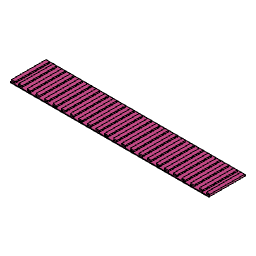
0_15m_Joch_Gerade_Schablone (Autodesk Fusion 360 design; units mm, degrees)
Autodesk Fusion 360 part; units mm, degrees
sketch "Skizze1" plane through (0, 0, 0) normal (0, 0, 1) x (1, 0, 0)
  line L0 (-3, 29.1) -> (3, 29.1)
  line L1 (3, 29.1) -> (3, 0)
  line L2 (3, 0) -> (-3, 0)
  line L3 (-3, 0) -> (-3, 29.1)
  line L4 (0, 29.1) -> (0, 0) construction
  line L5 (0, 0) -> (500, 0) construction
  line L6 (9.1, 29.1) -> (15.1, 29.1)
  line L7 (15.1, 29.1) -> (15.1, 0)
  line L8 (15.1, 0) -> (9.1, 0)
  line L9 (9.1, 0) -> (9.1, 29.1)
  line L10 (12.1, 29.1) -> (12.1, 0) construction
  line L11 (26.5, 29.1) -> (26.5, 0) construction
  line L12 (23.5, 29.1) -> (29.5, 29.1)
  line L13 (29.5, 0) -> (23.5, 0)
  line L14 (23.5, 0) -> (23.5, 29.1)
  line L15 (29.5, 29.1) -> (29.5, 0)
  line L16 (58.3, 0) -> (52.3, 0)
  line L17 (55.3, 29.1) -> (55.3, 0) construction
  line L18 (43.9, 29.1) -> (43.9, 0)
  line L19 (37.9, 29.1) -> (43.9, 29.1)
  line L20 (52.3, 29.1) -> (58.3, 29.1)
  line L21 (58.3, 29.1) -> (58.3, 0)
  line L22 (40.9, 29.1) -> (40.9, 0) construction
  line L23 (43.9, 0) -> (37.9, 0)
  line L24 (52.3, 0) -> (52.3, 29.1)
  line L25 (37.9, 0) -> (37.9, 29.1)
  line L26 (84.1, 29.1) -> (84.1, 0) construction
  line L27 (66.7, 0) -> (66.7, 29.1)
  line L28 (69.7, 29.1) -> (69.7, 0) construction
  line L29 (95.5, 0) -> (95.5, 29.1)
  line L30 (98.5, 29.1) -> (98.5, 0) construction
  line L31 (66.7, 29.1) -> (72.7, 29.1)
  line L32 (81.1, 0) -> (81.1, 29.1)
  line L33 (72.7, 29.1) -> (72.7, 0)
  line L34 (101.5, 29.1) -> (101.5, 0)
  line L35 (95.5, 29.1) -> (101.5, 29.1)
  line L36 (109.9, 29.1) -> (115.9, 29.1)
  line L37 (72.7, 0) -> (66.7, 0)
  line L38 (87.1, 0) -> (81.1, 0)
  line L39 (109.9, 0) -> (109.9, 29.1)
  line L40 (115.9, 0) -> (109.9, 0)
  line L41 (115.9, 29.1) -> (115.9, 0)
  line L42 (112.9, 29.1) -> (112.9, 0) construction
  line L43 (81.1, 29.1) -> (87.1, 29.1)
  line L44 (87.1, 29.1) -> (87.1, 0)
  line L45 (101.5, 0) -> (95.5, 0)
  line L46 (156.1, 29.1) -> (156.1, 0) construction
  line L47 (144.7, 29.1) -> (144.7, 0)
  line L48 (153.1, 29.1) -> (159.1, 29.1)
  line L49 (138.7, 29.1) -> (144.7, 29.1)
  line L50 (153.1, 0) -> (153.1, 29.1)
  line L51 (167.5, 29.1) -> (173.5, 29.1)
  line L52 (196.3, 0) -> (196.3, 29.1)
  line L53 (202.3, 0) -> (196.3, 0)
  line L54 (216.7, 0) -> (210.7, 0)
  line L55 (130.3, 29.1) -> (130.3, 0)
  line L56 (130.3, 0) -> (124.3, 0)
  line L57 (181.9, 29.1) -> (187.9, 29.1)
  line L58 (173.5, 29.1) -> (173.5, 0)
  line L59 (124.3, 0) -> (124.3, 29.1)
  line L60 (144.7, 0) -> (138.7, 0)
  line L61 (210.7, 0) -> (210.7, 29.1)
  line L62 (225.1, 29.1) -> (231.1, 29.1)
  line L63 (127.3, 29.1) -> (127.3, 0) construction
  line L64 (159.1, 29.1) -> (159.1, 0)
  line L65 (210.7, 29.1) -> (216.7, 29.1)
  line L66 (187.9, 0) -> (181.9, 0)
  line L67 (216.7, 29.1) -> (216.7, 0)
  line L68 (138.7, 0) -> (138.7, 29.1)
  line L69 (187.9, 29.1) -> (187.9, 0)
  line L70 (199.3, 29.1) -> (199.3, 0) construction
  line L71 (213.7, 29.1) -> (213.7, 0) construction
  line L72 (228.1, 29.1) -> (228.1, 0) construction
  line L73 (159.1, 0) -> (153.1, 0)
  line L74 (170.5, 29.1) -> (170.5, 0) construction
  line L75 (196.3, 29.1) -> (202.3, 29.1)
  line L76 (141.7, 29.1) -> (141.7, 0) construction
  line L77 (225.1, 0) -> (225.1, 29.1)
  line L78 (184.9, 29.1) -> (184.9, 0) construction
  line L79 (181.9, 0) -> (181.9, 29.1)
  line L80 (173.5, 0) -> (167.5, 0)
  line L81 (231.1, 29.1) -> (231.1, 0)
  line L82 (167.5, 0) -> (167.5, 29.1)
  line L83 (202.3, 29.1) -> (202.3, 0)
  line L84 (124.3, 29.1) -> (130.3, 29.1)
  line L85 (231.1, 0) -> (225.1, 0)
  line L86 (288.7, 29.1) -> (288.7, 0)
  line L87 (317.5, 0) -> (311.5, 0)
  line L88 (329.7, 29.1) -> (329.7, 0)
  line L89 (285.7, 29.1) -> (285.7, 0) construction
  line L90 (329.7, 0) -> (323.7, 0)
  line L91 (311.5, 29.1) -> (317.5, 29.1)
  line L92 (303.1, 29.1) -> (303.1, 0)
  line L93 (245.5, 0) -> (239.5, 0)
  line L94 (323.7, 29.1) -> (329.7, 29.1)
  line L95 (271.3, 29.1) -> (271.3, 0) construction
  line L96 (282.7, 29.1) -> (288.7, 29.1)
  line L97 (282.7, 0) -> (282.7, 29.1)
  line L98 (300.1, 29.1) -> (300.1, 0) construction
  line L99 (274.3, 29.1) -> (274.3, 0)
  line L100 (326.7, 29.1) -> (326.7, 0) construction
  line L101 (268.3, 0) -> (268.3, 29.1)
  line L102 (259.9, 0) -> (253.9, 0)
  line L103 (253.9, 29.1) -> (259.9, 29.1)
  line L104 (303.1, 0) -> (297.1, 0)
  line L105 (288.7, 0) -> (282.7, 0)
  line L106 (297.1, 29.1) -> (303.1, 29.1)
  line L107 (314.5, 29.1) -> (314.5, 0) construction
  line L108 (317.5, 29.1) -> (317.5, 0)
  line L109 (245.5, 29.1) -> (245.5, 0)
  line L110 (323.7, 0) -> (323.7, 29.1)
  line L111 (239.5, 29.1) -> (245.5, 29.1)
  line L112 (253.9, 0) -> (253.9, 29.1)
  line L113 (239.5, 0) -> (239.5, 29.1)
  line L114 (242.5, 29.1) -> (242.5, 0) construction
  line L115 (311.5, 0) -> (311.5, 29.1)
  line L116 (259.9, 29.1) -> (259.9, 0)
  line L117 (268.3, 29.1) -> (274.3, 29.1)
  line L118 (274.3, 0) -> (268.3, 0)
  line L119 (297.1, 0) -> (297.1, 29.1)
  line L120 (256.9, 29.1) -> (256.9, 0) construction
  dimension "d3" = 500
  dimension "d4" = 29.1
  dimension "d5" = 6
  dimension "d8" = 29.1
  dimension "d9" = 6
  dimension "d10" = 29.1
  dimension "d11" = 6
  dimension "d12" = 29.1
  dimension "d13" = 6
  dimension "d14" = 29.1
  dimension "d15" = 6
  dimension "d16" = 29.1
  dimension "d17" = 6
  dimension "d18" = 29.1
  dimension "d19" = 6
  dimension "d20" = 29.1
  dimension "d21" = 6
  dimension "d22" = 29.1
  dimension "d23" = 6
  dimension "d24" = 29.1
  dimension "d25" = 6
  dimension "d26" = 29.1
  dimension "d27" = 6
  dimension "d28" = 29.1
  dimension "d29" = 6
  dimension "d30" = 29.1
  dimension "d31" = 6
  dimension "d32" = 29.1
  dimension "d33" = 6
  dimension "d34" = 29.1
  dimension "d35" = 6
  dimension "d36" = 29.1
  dimension "d37" = 6
  dimension "d38" = 29.1
  dimension "d39" = 6
  dimension "d40" = 29.1
  dimension "d41" = 6
  dimension "d42" = 29.1
  dimension "d43" = 6
  dimension "d44" = 29.1
  dimension "d45" = 6
  dimension "d46" = 29.1
  dimension "d47" = 6
  dimension "d48" = 29.1
  dimension "d49" = 6
  dimension "d50" = 29.1
  dimension "d51" = 6
  dimension "d52" = 29.1
  dimension "d53" = 6
  dimension "d54" = 12.1
  dimension "d55" = 14.4
  dimension "d56" = 14.4
  dimension "d57" = 14.4
  dimension "d58" = 14.4
  dimension "d59" = 14.4
  dimension "d60" = 14.4
  dimension "d61" = 14.4
  dimension "d62" = 14.4
  dimension "d63" = 14.4
  dimension "d64" = 14.4
  dimension "d65" = 14.4
  dimension "d66" = 14.4
  dimension "d67" = 14.4
  dimension "d68" = 14.4
  dimension "d69" = 14.4
  dimension "d70" = 14.4
  dimension "d71" = 14.4
  dimension "d72" = 14.4
  dimension "d73" = 14.4
  dimension "d74" = 14.4
  dimension "d75" = 14.4
  dimension "d76" = 12.2
  constraint horizontal L0
  constraint vertical L1
  constraint horizontal L2
  constraint vertical L3
  constraint midpoint L0 L4.start
  constraint midpoint L2 L4.end
  constraint coincident L4.end L5.start
  constraint perpendicular L4 L5
  constraint horizontal L6
  constraint vertical L7
  constraint horizontal L8
  constraint vertical L9
  constraint midpoint L6 L10.start
  constraint midpoint L8 L10.end
  constraint horizontal L12
  constraint vertical L15
  constraint horizontal L13
  constraint vertical L14
  constraint midpoint L11.start L12
  constraint midpoint L11.end L13
  constraint horizontal L19
  constraint vertical L18
  constraint horizontal L23
  constraint vertical L25
  constraint midpoint L22.start L19
  constraint midpoint L22.end L23
  constraint horizontal L20
  constraint vertical L21
  constraint horizontal L16
  constraint vertical L24
  constraint midpoint L17.start L20
  constraint midpoint L17.end L16
  constraint horizontal L31
  constraint vertical L33
  constraint horizontal L37
  constraint vertical L27
  constraint midpoint L28.start L31
  constraint midpoint L28.end L37
  constraint horizontal L43
  constraint vertical L44
  constraint horizontal L38
  constraint vertical L32
  constraint midpoint L26.start L43
  constraint midpoint L26.end L38
  constraint horizontal L35
  constraint vertical L34
  constraint horizontal L45
  constraint vertical L29
  constraint midpoint L30.start L35
  constraint midpoint L30.end L45
  constraint horizontal L36
  constraint vertical L41
  constraint horizontal L40
  constraint vertical L39
  constraint midpoint L42.start L36
  constraint midpoint L42.end L40
  constraint horizontal L84
  constraint vertical L55
  constraint horizontal L56
  constraint vertical L59
  constraint midpoint L63.start L84
  constraint midpoint L63.end L56
  constraint horizontal L49
  constraint vertical L47
  constraint horizontal L60
  constraint vertical L68
  constraint midpoint L76.start L49
  constraint midpoint L76.end L60
  constraint horizontal L48
  constraint vertical L64
  constraint horizontal L73
  constraint vertical L50
  constraint midpoint L46.start L48
  constraint midpoint L46.end L73
  constraint horizontal L51
  constraint vertical L58
  constraint horizontal L80
  constraint vertical L82
  constraint midpoint L74.start L51
  constraint midpoint L74.end L80
  constraint horizontal L57
  constraint vertical L69
  constraint horizontal L66
  constraint vertical L79
  constraint midpoint L78.start L57
  constraint midpoint L78.end L66
  constraint horizontal L75
  constraint vertical L83
  constraint horizontal L53
  constraint vertical L52
  constraint midpoint L70.start L75
  constraint midpoint L70.end L53
  constraint horizontal L65
  constraint vertical L67
  constraint horizontal L54
  constraint vertical L61
  constraint midpoint L71.start L65
  constraint midpoint L71.end L54
  constraint horizontal L62
  constraint vertical L81
  constraint horizontal L85
  constraint vertical L77
  constraint midpoint L72.start L62
  constraint midpoint L72.end L85
  constraint horizontal L111
  constraint vertical L109
  constraint horizontal L93
  constraint vertical L113
  constraint midpoint L114.start L111
  constraint midpoint L114.end L93
  constraint horizontal L103
  constraint vertical L116
  constraint horizontal L102
  constraint vertical L112
  constraint midpoint L120.start L103
  constraint midpoint L120.end L102
  constraint horizontal L117
  constraint vertical L99
  constraint horizontal L118
  constraint vertical L101
  constraint midpoint L95.start L117
  constraint midpoint L95.end L118
  constraint horizontal L96
  constraint vertical L86
  constraint horizontal L105
  constraint vertical L97
  constraint midpoint L89.start L96
  constraint midpoint L89.end L105
  constraint horizontal L106
  constraint vertical L92
  constraint horizontal L104
  constraint vertical L119
  constraint midpoint L98.start L106
  constraint midpoint L98.end L104
  constraint horizontal L91
  constraint vertical L108
  constraint horizontal L87
  constraint vertical L115
  constraint midpoint L107.start L91
  constraint midpoint L107.end L87
  constraint horizontal L94
  constraint vertical L88
  constraint horizontal L90
  constraint vertical L110
  constraint midpoint L100.start L94
  constraint midpoint L100.end L90
  constraint coincident L5 L10.end
  constraint coincident L5 L11.end
  constraint coincident L5 L22.end
  constraint coincident L5 L17.end
  constraint coincident L5 L28.end
  constraint coincident L5 L26.end
  constraint coincident L5 L30.end
  constraint coincident L5 L42.end
  constraint coincident L5 L63.end
  constraint coincident L5 L76.end
  constraint coincident L5 L46.end
  constraint coincident L5 L74.end
  constraint coincident L5 L78.end
  constraint coincident L5 L70.end
  constraint coincident L5 L71.end
  constraint coincident L5 L72.end
  constraint coincident L5 L114.end
  constraint coincident L5 L120.end
  constraint coincident L5 L95.end
  constraint coincident L5 L89.end
  constraint coincident L5 L98.end
  constraint coincident L5 L107.end
  constraint coincident L5 L100.end
  measures "d3" distance of L4.end L5.end
  measures "d4" distance of L0 L2
  measures "d5" distance of L1 L3
  measures "d8" distance of L6 L8
  measures "d9" distance of L7 L9
  measures "d10" distance of L12 L13
  measures "d11" distance of L14 L15
  measures "d12" distance of L19 L23
  measures "d13" distance of L18 L25
  measures "d14" distance of L16 L20
  measures "d15" distance of L21 L24
  measures "d16" distance of L31 L37
  measures "d17" distance of L27 L33
  measures "d18" distance of L38 L43
  measures "d19" distance of L32 L44
  measures "d20" distance of L35 L45
  measures "d21" distance of L29 L34
  measures "d22" distance of L36 L40
  measures "d23" distance of L39 L41
  measures "d24" distance of L56 L84
  measures "d25" distance of L55 L59
  measures "d26" distance of L49 L60
  measures "d27" distance of L47 L68
  measures "d28" distance of L48 L73
  measures "d29" distance of L50 L64
  measures "d30" distance of L51 L80
  measures "d31" distance of L58 L82
  measures "d32" distance of L57 L66
  measures "d33" distance of L69 L79
  measures "d34" distance of L53 L75
  measures "d35" distance of L52 L83
  measures "d36" distance of L54 L65
  measures "d37" distance of L61 L67
  measures "d38" distance of L62 L85
  measures "d39" distance of L77 L81
  measures "d40" distance of L93 L111
  measures "d41" distance of L109 L113
  measures "d42" distance of L102 L103
  measures "d43" distance of L112 L116
  measures "d44" distance of L117 L118
  measures "d45" distance of L99 L101
  measures "d46" distance of L96 L105
  measures "d47" distance of L86 L97
  measures "d48" distance of L104 L106
  measures "d49" distance of L92 L119
  measures "d50" distance of L87 L91
  measures "d51" distance of L108 L115
  measures "d52" distance of L90 L94
  measures "d53" distance of L88 L110
  measures "d54" distance of L4 L10
  measures "d55" distance of L10 L11
  measures "d56" distance of L11 L22
  measures "d57" distance of L17 L22
  measures "d58" distance of L17 L28
  measures "d59" distance of L26 L28
  measures "d60" distance of L26 L30
  measures "d61" distance of L30 L42
  measures "d62" distance of L42 L63
  measures "d63" distance of L63 L76
  measures "d64" distance of L46 L76
  measures "d65" distance of L46 L74
  measures "d66" distance of L74 L78
  measures "d67" distance of L70 L78
  measures "d68" distance of L70 L71
  measures "d69" distance of L71 L72
  measures "d70" distance of L72 L114
  measures "d71" distance of L114 L120
  measures "d72" distance of L95 L120
  measures "d73" distance of L89 L95
  measures "d74" distance of L89 L98
  measures "d75" distance of L98 L107
  measures "d76" distance of L100 L107
extrude "Extrusion1" add sketch "Skizze1" along normal blind 3 makes body 1 at (301.1, 19.4, 0) makes body 2 at (243.5, 9.7, 0) makes body 3 at (183.9, 19.4, 0) makes body 4 at (126.3, 9.7, 0) makes body 5 at (68.7, 19.4, 0) makes body 6 at (13.1, 9.7, 0) makes body 7 at (27.5, 9.7, 0) makes body 8 at (83.1, 9.7, 0) makes body 9 at (140.7, 19.4, 0) makes body 10 at (200.3, 9.7, 0) makes body 11 at (255.9, 9.7, 0) makes body 12 at (313.5, 9.7, 0) makes body 13 at (284.7, 9.7, 0) makes body 14 at (229.1, 9.7, 0) makes body 15 at (171.5, 9.7, 0) makes body 16 at (113.9, 19.4, 0) makes body 17 at (56.3, 9.7, 0) makes body 18 at (1, 9.7, 0) makes body 19 at (41.9, 9.7, 0) makes body 20 at (97.5, 9.7, 0) makes body 21 at (155.1, 19.4, 0) makes body 22 at (212.7, 19.4, 0) makes body 23 at (270.3, 9.7, 0) makes body 24 at (327.7, 19.4, 0)
move_face "Flächen versetzen1" offset 29.1 24 faces at (229.1, 0, 1) (56.3, 0, 1) (1, 0, 1) (41.9, 0, 1) (99.5, 0, 1) (157.1, 0, 1) (214.7, 0, 1) (272.3, 0, 1) (327.7, 0, 1) (286.7, 0, 1) (301.1, 0, 1) (243.5, 0, 1) (185.9, 0, 1) (128.3, 0, 1) (70.7, 0, 1) (13.1, 0, 1) (27.5, 0, 1) (85.1, 0, 1) (142.7, 0, 1) (200.3, 0, 1) (257.9, 0, 1) (315.5, 0, 1) (171.5, 0, 1) (113.9, 0, 1) on bodies 1 2 3 4 5 6 7 8 9 10 11 12 13 14 15 16 17 18 19 20 21 22 23 24
sketch "Skizze2" plane through (0, 0, 0) normal (0, 0, 1) x (1, 0, 0)
  line L0 (-3, 29.1) -> (-3, -29.1)
  line L1 (329.7, -29.1) -> (329.7, 29.1)
  line L2 (-3, 29.1) -> (-3, 31.1)
  line L3 (-3, -29.1) -> (-3, -31.1)
  line L4 (329.7, 29.1) -> (329.7, 31.1)
  line L5 (329.7, -29.1) -> (329.7, -31.1)
  line L6 (-3, 31.1) -> (329.7, 31.1)
  line L7 (-3, -31.1) -> (329.7, -31.1)
  dimension "d80" = 2
  dimension "d81" = 2
  dimension "d82" = 2
  dimension "d83" = 2
  constraint coincident L0.start L2.start
  constraint coincident L0.end L3.start
  constraint coincident L1.end L4.start
  constraint coincident L1.start L5.start
  constraint parallel L0 L2
  constraint parallel L0 L3
  constraint parallel L1 L5
  constraint parallel L1 L4
  measures "d80" distance of L0.start L2.end
  measures "d81" distance of L0.end L3.end
  measures "d82" distance of L1.end L4.end
  measures "d83" distance of L1.start L5.end
extrude "Extrusion2" add sketch "Skizze2" along normal blind 1 separate body makes body 25
combine "Kombinieren1" operation cut target body 25 tool bodies 18 6 7 19 17 5 8 20 16 4 9 21 15 3 10 22 14 2 11 23 13 1 12 24 keep tools
equation "Schwellen_Länge = 58 mm + 0.2 mm"
equation "Schwellen_Breite = 5.8 mm + 0.2 mm"
equation "d4 = Schwellen_Länge / 2"
equation "d5 = Schwellen_Breite"
equation "d8 = Schwellen_Länge / 2"
equation "d9 = Schwellen_Breite"
equation "d10 = Schwellen_Länge / 2"
equation "d11 = Schwellen_Breite"
equation "d12 = Schwellen_Länge / 2"
equation "d13 = Schwellen_Breite"
equation "d14 = Schwellen_Länge / 2"
equation "d15 = Schwellen_Breite"
equation "d16 = Schwellen_Länge / 2"
equation "d17 = Schwellen_Breite"
equation "d18 = Schwellen_Länge / 2"
equation "d19 = Schwellen_Breite"
equation "d20 = Schwellen_Länge / 2"
equation "d21 = Schwellen_Breite"
equation "d22 = Schwellen_Länge / 2"
equation "d23 = Schwellen_Breite"
equation "d24 = Schwellen_Länge / 2"
equation "d25 = Schwellen_Breite"
equation "d26 = Schwellen_Länge / 2"
equation "d27 = Schwellen_Breite"
equation "d28 = Schwellen_Länge / 2"
equation "d29 = Schwellen_Breite"
equation "d30 = Schwellen_Länge / 2"
equation "d31 = Schwellen_Breite"
equation "d32 = Schwellen_Länge / 2"
equation "d33 = Schwellen_Breite"
equation "d34 = Schwellen_Länge / 2"
equation "d35 = Schwellen_Breite"
equation "d36 = Schwellen_Länge / 2"
equation "d37 = Schwellen_Breite"
equation "d38 = Schwellen_Länge / 2"
equation "d39 = Schwellen_Breite"
equation "d40 = Schwellen_Länge / 2"
equation "d41 = Schwellen_Breite"
equation "d42 = Schwellen_Länge / 2"
equation "d43 = Schwellen_Breite"
equation "d44 = Schwellen_Länge / 2"
equation "d45 = Schwellen_Breite"
equation "d46 = Schwellen_Länge / 2"
equation "d47 = Schwellen_Breite"
equation "d48 = Schwellen_Länge / 2"
equation "d49 = Schwellen_Breite"
equation "d50 = Schwellen_Länge / 2"
equation "d51 = Schwellen_Breite"
equation "d52 = Schwellen_Länge / 2"
equation "d53 = Schwellen_Breite"
equation "d54 = Schwellen_Abstand_Anfang"
equation "d55 = Schwellen_Abstand_Mitte"
equation "d56 = Schwellen_Abstand_Mitte"
equation "d57 = Schwellen_Abstand_Mitte"
equation "d58 = Schwellen_Abstand_Mitte"
equation "d59 = Schwellen_Abstand_Mitte"
equation "d60 = Schwellen_Abstand_Mitte"
equation "d61 = Schwellen_Abstand_Mitte"
equation "d62 = Schwellen_Abstand_Mitte"
equation "d63 = Schwellen_Abstand_Mitte"
equation "d64 = Schwellen_Abstand_Mitte"
equation "d65 = Schwellen_Abstand_Mitte"
equation "d66 = Schwellen_Abstand_Mitte"
equation "d67 = Schwellen_Abstand_Mitte"
equation "d68 = Schwellen_Abstand_Mitte"
equation "d69 = Schwellen_Abstand_Mitte"
equation "d70 = Schwellen_Abstand_Mitte"
equation "d71 = Schwellen_Abstand_Mitte"
equation "d72 = Schwellen_Abstand_Mitte"
equation "d73 = Schwellen_Abstand_Mitte"
equation "d74 = Schwellen_Abstand_Mitte"
equation "d75 = Schwellen_Abstand_Mitte"
equation "d76 = Schwellen_Abstand_Ende"
equation "d79 = Schwellen_Länge / 2"
equation "d81 = d80"
equation "d82 = d80"
equation "d83 = d80"
equation "Schwellen_Abstand_Anfang = 12.1 mm"
equation "Schwellen_Abstand_Mitte = 14.4 mm"
equation "Schwellen_Abstand_Ende = 12.2 mm"
